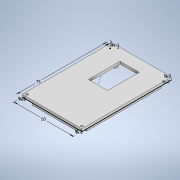
# Autodesk Inventor part: Enclosure Lid
Saved by Autodesk Inventor 2020.2 (Build 242310000, 310)
## iProperties
Created: 2020-09-23
Part Number: Enclosure Lid
Material: Generic
Document SubType Name: Modeling
Designer: johnf
Density: 1 g/cm^3
Appearance: Default
Author: johnf
Autodesk Inventor part; units mm, degrees
ref_plane "YZ Plane" through (0, 0, 0) normal (1, 0, 0) x (0, 1, 0)
ref_plane "XZ Plane" through (0, 0, 0) normal (0, 1, 0) x (-1, 0, 0)
ref_plane "XY Plane" through (0, 0, 0) normal (0, 0, 1) x (1, 0, 0)
sketch "Sketch1" plane through (0, 0, 0) normal (0, 1, 0) x (-1, 0, 0)
  line L0 (25, 37.5) -> (-25, 37.5)
  line L1 (-25, 37.5) -> (-25, -37.5)
  line L2 (-25, -37.5) -> (25, -37.5)
  line L3 (25, -37.5) -> (25, 37.5)
  line L4 (-25, 37.5) -> (25, -37.5) construction
  circle A0 centre (23, -35.5) radius 1
  circle A1 centre (-23, -35.5) radius 1
  circle A2 centre (-23, 35.5) radius 1
  circle A3 centre (23, 35.5) radius 1
  point P0 (0, 0)
  point P1 (0, 0)
  dimension "d0" = 75
  dimension "d1" = 50
  dimension "d17" = 2
  dimension "d18" = 2
  dimension "d21" = 2
  dimension "d22" = 2
  dimension "d23" = 2
  dimension "d25" = 2
  dimension "d26" = 2
  dimension "d27" = 2
  dimension "d28" = 2
  constraints: 10 end point, 4 centre point, 3 equal radius, 2 parallel, 1 coincident, 1 horizontal, 1 midpoint, 1 perpendicular
  measures "d0" distance of L2.end L0.start
  measures "d1" distance of L0.start L0.end
  measures "d17" distance from line of L2 A0.centre
  measures "d18" distance from line of A0.centre L3
  measures "d21" diameter of A0
  measures "d22" distance from line of A3.centre L0
  measures "d23" distance from line of L3 A3.centre
  measures "d25" distance from line of L0 A2.centre
  measures "d26" distance from line of L1 A2.centre
  measures "d27" distance from line of L1 A1.centre
  measures "d28" distance from line of L2 A1.centre
extrude "Extrusion1" add sketch "Sketch1" along normal blind 2
sketch "Sketch4" plane through (0, 0, 0) normal (0, -1, 0) x (1, 0, 0)
  line L0 (-18.8, 35.3) -> (18.8, 35.3)
  line L1 (22.8, 31.3) -> (22.8, -31.3)
  line L2 (18.8, -35.3) -> (-18.8, -35.3)
  line L3 (-22.8, -31.3) -> (-22.8, 31.3)
  line L4 (-22.8, 35.3) -> (22.8, -35.3) construction
  line L5 (-25, -37.5) -> (-25, 37.5) projected
  line L6 (-25, 37.5) -> (25, 37.5) projected
  arc A0 (-22.8, 31.3) -> (-18.8, 35.3) centre (-22.8, 35.3) ccw
  arc A1 (18.8, 35.3) -> (22.8, 31.3) centre (22.8, 35.3) ccw
  arc A2 (-18.8, -35.3) -> (-22.8, -31.3) centre (-22.8, -35.3) ccw
  arc A3 (22.8, -31.3) -> (18.8, -35.3) centre (22.8, -35.3) ccw
  line L7 (17.1431, 33.3) -> (-17.1431, 33.3)
  arc A4 (-20.8, 29.6431) -> (-17.1431, 33.3) centre (-22.8, 35.3) ccw
  line L8 (-20.8, 29.6431) -> (-20.8, -29.6431)
  arc A5 (-17.1431, -33.3) -> (-20.8, -29.6431) centre (-22.8, -35.3) ccw
  line L9 (-17.1431, -33.3) -> (17.1431, -33.3)
  arc A6 (20.8, -29.6431) -> (17.1431, -33.3) centre (22.8, -35.3) ccw
  line L10 (20.8, -29.6431) -> (20.8, 29.6431)
  arc A7 (17.1431, 33.3) -> (20.8, 29.6431) centre (22.8, 35.3) ccw
  point P0 (0, 0)
  point P1 (0, 0)
  dimension "d29" = 2.2
  dimension "d30" = 2.2
  dimension "d32" = 4
  dimension "d35" = 2
  constraints: 18 end point, 16 point on circle, 8 centre point, 8 point on line, 4 parallel, 3 coincident, 3 equal radius, 2 perpendicular, 1 horizontal, 1 midpoint, 7 other
  measures "d29" distance between parallel lines of L5 L3
  measures "d30" distance between parallel lines of L6 L0
  measures "d32" radius of A1
  measures "d35" distance between parallel lines of L0 L7
extrude "Extrusion4" add sketch "Sketch4" along normal blind 4
sketch "Sketch5" plane through (0, 0, 0) normal (0, -1, 0) x (1, 0, 0)
  line L0 (-10.4342, -25.835) -> (12.5658, -25.835) construction
  line L1 (12.5658, -25.835) -> (12.5658, -2.585) construction
  line L2 (12.5658, -2.585) -> (-10.4342, -2.585) construction
  line L3 (-10.4342, -2.585) -> (-10.4342, -25.835) construction
  line L4 (-10.4342, -2.585) -> (12.5658, -25.835) construction
  circle A0 centre (-10.4342, -2.585) radius 1
  circle A1 centre (-10.4342, -25.835) radius 1
  circle A2 centre (12.5658, -25.835) radius 1
  circle A3 centre (12.5658, -2.585) radius 1
  circle A4 centre (-10.4342, -25.835) radius 2
  circle A5 centre (-10.4342, -2.585) radius 2
  circle A6 centre (12.5658, -2.585) radius 2
  circle A7 centre (12.5658, -25.835) radius 2
  line L5 (-10.4342, -14.21) -> (12.5658, -14.21) construction
  point P0 (0, 0)
  dimension "d36" = 23.25
  dimension "d37" = 23
  dimension "d38" = 2
  dimension "d39" = 4
  constraints: 12 end point, 8 centre point, 8 coincident, 6 equal radius, 2 midpoint, 2 parallel, 1 horizontal, 1 perpendicular
  measures "d36" distance of L2.end L0.start
  measures "d37" distance of L0.start L0.end
  measures "d38" diameter of A0
  measures "d39" diameter of A4
extrude "Extrusion5" add sketch "Sketch5" along normal blind 2
sketch "Sketch6" plane through (0, 0, 0) normal (0, -1, 0) x (1, 0, 0)
  line L0 (-7.9342, -27.46) -> (8.0658, -27.46)
  line L1 (8.0658, -27.46) -> (8.0658, -0.96)
  line L2 (8.0658, -0.96) -> (-7.9342, -0.96)
  line L3 (-7.9342, -0.96) -> (-7.9342, -27.46)
  circle A0 centre (-10.4342, -25.835) radius 1 projected
  line L4 (-10.58, -24.8457) -> (-10.58, -3.5743) construction
  circle A1 centre (-10.4342, -2.585) radius 1 projected
  line L5 (-10.58, -14.21) -> (-1.6995, -14.21) construction
  point P0 (0, 0)
  dimension "d42" = 16
  dimension "d43" = 26.5
  dimension "d45" = 1.5
  constraints: 12 end point, 2 parallel, 1 horizontal, 1 midpoint, 1 perpendicular, 1 vertical, 5 other
  measures "d42" distance of L0.start L0.end
  measures "d43" distance of L2.end L0.start
extrude "Extrusion6" cut sketch "Sketch6" against normal blind 10 contours L3 L2 L1 L0
equation "\"d18\" = d17"
equation "\"d22\" = d17"
equation "\"d23\" = d17"
equation "\"d25\" = d17"
equation "\"d26\" = d17"
equation "\"d27\" = d17"
equation "\"d28\" = d17"
equation "\"d30\" = d29"
body "Solid1"
